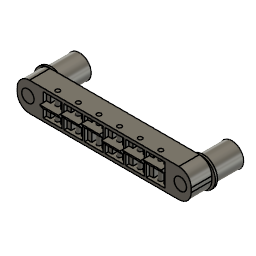
logo metal_ (Autodesk Fusion 360 archive; units mm, degrees)
design "Most Gotoh"
part number: 2026-09-04-10-43-11-082
Autodesk Fusion 360 part; units mm, degrees
note: some values were not read from the file. Chosen so that the rebuilt part matches the saved one: which bodies a step acts on; which face or edge a step refers to.
sketch "Szkic1" plane through (0, 0, 0) normal (0, 0, 1) x (1, 0, 0)
  line L0 (0, 0) -> (74, 0) construction
  circle A0 centre (0, 0) radius 3
  circle A1 centre (74, 0) radius 3
  line L1 (73.25, 7) -> (0.75, 7)
  line L2 (-5.25, 1) -> (-5.25, -1)
  line L3 (0.75, -7) -> (73.25, -7)
  line L4 (79.25, -1) -> (79.25, 1)
  line L5 (37, 5.5) -> (37, -5.5) construction
  line L6 (36.5, 5.5) -> (36.5, -5.5)
  line L7 (37.5, 5.5) -> (37.5, -5.5)
  line L8 (46.5, 5.5) -> (46.5, -5.5)
  line L9 (39.5, 5.5) -> (39.5, -5.5)
  line L10 (44.5, 5.5) -> (44.5, -5.5)
  line L11 (54.5, 5.5) -> (54.5, -5.5)
  line L12 (56.5, 5.5) -> (56.5, -5.5)
  line L13 (49.5, 5.5) -> (49.5, -5.5)
  line L14 (47.5, 5.5) -> (47.5, -5.5)
  line L15 (59.5, 5.5) -> (59.5, -5.5)
  line L16 (64.5, 5.5) -> (64.5, -5.5)
  line L17 (66.5, 5.5) -> (66.5, -5.5)
  line L18 (57.5, 5.5) -> (57.5, -5.5)
  line L19 (24.5, 5.5) -> (24.5, -5.5)
  line L20 (17.5, 5.5) -> (17.5, -5.5)
  line L21 (34.5, 5.5) -> (34.5, -5.5)
  line L22 (26.5, 5.5) -> (26.5, -5.5)
  line L23 (27.5, 5.5) -> (27.5, -5.5)
  line L24 (36.5, 5.5) -> (36.5, -5.5)
  line L25 (19.5, 5.5) -> (19.5, -5.5)
  line L26 (16.5, 5.5) -> (16.5, -5.5)
  line L27 (7.5, 5.5) -> (7.5, -5.5)
  line L28 (29.5, 5.5) -> (29.5, -5.5)
  line L29 (9.5, 5.5) -> (9.5, -5.5)
  line L30 (14.5, 5.5) -> (14.5, -5.5)
  arc A2 (79.25, 1) -> (73.25, 7) centre (73.25, 1) ccw
  arc A3 (73.25, -7) -> (79.25, -1) centre (73.25, -1) ccw
  arc A4 (-5.25, -1) -> (0.75, -7) centre (0.75, -1) ccw
  arc A5 (0.75, 7) -> (-5.25, 1) centre (0.75, 1) ccw
  line L31 (66.5, 5.5) -> (7.5, 5.5)
  line L32 (7.5, -5.5) -> (66.5, -5.5)
  point P0 (-5.25, 7)
  point P1 (-5.25, -7)
  point P2 (79.25, -7)
  point P3 (37, 0)
  dimension "d1" = 74
  dimension "d2" = 6
  dimension "d3" = 6
  dimension "d4" = 84.5
  dimension "d5" = 14
  dimension "d15" = -2
  dimension "d16" = 2
  dimension "d17" = -9
  dimension "d18" = -2
  dimension "d19" = 2
  dimension "d20" = -9
  dimension "d21" = -2
  dimension "d22" = 2
  dimension "d23" = 6
  dimension "d24" = 6
  constraint coincident L0.start A0.centre
  constraint horizontal L0
  constraint coincident L0.end A1.centre
  constraint perpendicular L1 L2
  constraint parallel L1 L3
  constraint parallel L2 L4
  constraint midpoint L0 P3
  constraint coincident L7.start L31
  constraint coincident L6.start L31
  constraint coincident L7.end L32
  constraint coincident L6.end L32
  constraint coincident L5.end L32
  constraint coincident L5.start L31
  constraint symmetric L5 L7.start L6.start
  constraint symmetric L5 L7.end L6.end
  constraint symmetric L5 L8.start L23.start
  constraint symmetric L5 L8.end L23.end
  constraint symmetric L5 L9.start L21.start
  constraint symmetric L5 L9.end L21.end
  constraint symmetric L5 L10.start L28.start
  constraint symmetric L5 L10.end L28.end
  constraint symmetric L5 L13.end L19.end
  constraint symmetric L5 L13.start L19.start
  constraint symmetric L5 L11.end L25.end
  constraint symmetric L5 L11.start L25.start
  constraint symmetric L5 L12.start L20.start
  constraint symmetric L5 L12.end L20.end
  constraint symmetric L5 L14.start L22.start
  constraint symmetric L5 L14.end L22.end
  constraint symmetric L5 L15.end L30.end
  constraint symmetric L5 L15.start L30.start
  constraint symmetric L5 L16.end L29.end
  constraint symmetric L5 L18.end L26.end
  constraint symmetric L5 L17.end L27.end
  constraint symmetric L5 L17.start L27.start
  constraint symmetric L5 L16.start L29.start
  constraint symmetric L5 L18.start L26.start
  constraint tangent L1 A2
  constraint tangent L4 A2
  constraint coincident P2 L4
  constraint coincident P2 L3
  constraint tangent L4 A3
  constraint tangent L3 A3
  constraint equal A2 A3
  constraint coincident P1 L3
  constraint coincident P1 L2
  constraint tangent L3 A4
  constraint tangent L2 A4
  constraint equal A2 A4
  constraint coincident P0 L1
  constraint coincident P0 L2
  constraint tangent L1 A5
  constraint tangent L2 A5
  measures "d1" distance of L0.start L0.end
  measures "d2" diameter of A0
  measures "d3" diameter of A1
  measures "d4" distance of P1 P2
  measures "d5" distance of P0 P1
  measures "d23" radius of A2
  measures "d24" radius of A5
extrude "Wyciągnięcie proste1" add sketch "Szkic1" against normal blind 10 contours L1 L2 L3 L4 A2 A3 A4 A5 | L6 L7 L24 L31 L32 | L6 L21 L24 L31 L32 | L7 L9 L31 L32 | L21 L28 L31 L32 | L9 L10 L31 L32 | L23 L28 L31 L32 | L8 L10 L31 L32 | L22 L23 L31 L32 | L8 L14 L31 L32 | L19 L22 L31 L32 | L13 L14 L31 L32 | L19 L25 L31 L32 | L11 L13 L31 L32 | L20 L25 L31 L32 | L11 L12 L31 L32 | L20 L26 L31 L32 | L12 L18 L31 L32 | L26 L30 L31 L32 | L15 L18 L31 L32 | L29 L30 L31 L32 | L15 L16 L31 L32 | L27 L29 L31 L32 | L16 L17 L31 L32 makes body 1
extrude "Wyciągnięcie proste2" cut sketch "Szkic1" against normal blind 8 contours L21 L28 L31 L32 | L9 L10 L31 L32 | L19 L25 L31 L32 | L11 L13 L31 L32 | L29 L30 L31 L32 | L15 L16 L31 L32 bodies 1
extrude "Wyciągnięcie proste3" cut sketch "Szkic1" against normal blind 1.5 contours L6 L21 L24 L31 L32 | L7 L9 L31 L32 | L23 L28 L31 L32 | L8 L10 L31 L32 | L19 L22 L31 L32 | L13 L14 L31 L32 | L20 L25 L31 L32 | L11 L12 L31 L32 | L26 L30 L31 L32 | L15 L18 L31 L32 | L27 L29 L31 L32 | L16 L17 L31 L32 bodies 1
sketch "Szkic2" plane through (0, -7, 0) normal (0, -1, 0) x (1, 0, 0)
  line L0 (73.25, 0) -> (0.75, 0)
  line L1 (0.75, 0) -> (0.75, -10)
  line L2 (0.75, -10) -> (73.25, -10)
  line L3 (73.25, -10) -> (73.25, 0)
  line L4 (37, 0) -> (37, -10)
  line L5 (27.5, 0) -> (36.5, 0)
  line L6 (36.5, 0) -> (36.5, -1.5)
  line L7 (36.5, -1.5) -> (34.5, -1.5)
  line L8 (34.5, -1.5) -> (34.5, -8)
  line L9 (34.5, -8) -> (29.5, -8)
  line L10 (29.5, -8) -> (29.5, -1.5)
  line L11 (29.5, -1.5) -> (27.5, -1.5)
  line L12 (27.5, -1.5) -> (27.5, 0)
  line L13 (17.5, 0) -> (26.5, 0)
  line L14 (26.5, 0) -> (26.5, -1.5)
  line L15 (26.5, -1.5) -> (24.5, -1.5)
  line L16 (24.5, -1.5) -> (24.5, -8)
  line L17 (24.5, -8) -> (19.5, -8)
  line L18 (19.5, -8) -> (19.5, -1.5)
  line L19 (19.5, -1.5) -> (17.5, -1.5)
  line L20 (17.5, -1.5) -> (17.5, 0)
  line L21 (7.5, 0) -> (16.5, 0)
  line L22 (16.5, 0) -> (16.5, -1.5)
  line L23 (16.5, -1.5) -> (14.5, -1.5)
  line L24 (14.5, -1.5) -> (14.5, -8)
  line L25 (14.5, -8) -> (9.5, -8)
  line L26 (9.5, -8) -> (9.5, -1.5)
  line L27 (9.5, -1.5) -> (7.5, -1.5)
  line L28 (7.5, -1.5) -> (7.5, 0)
  line L29 (37.5, 0) -> (46.5, 0)
  line L30 (46.5, 0) -> (46.5, -1.5)
  line L31 (46.5, -1.5) -> (44.5, -1.5)
  line L32 (44.5, -1.5) -> (44.5, -8)
  line L33 (44.5, -8) -> (39.5, -8)
  line L34 (39.5, -8) -> (39.5, -1.5)
  line L35 (39.5, -1.5) -> (37.5, -1.5)
  line L36 (37.5, -1.5) -> (37.5, 0)
  line L37 (47.5, 0) -> (56.5, 0)
  line L38 (56.5, 0) -> (56.5, -1.5)
  line L39 (56.5, -1.5) -> (54.5, -1.5)
  line L40 (54.5, -1.5) -> (54.5, -8)
  line L41 (54.5, -8) -> (49.5, -8)
  line L42 (49.5, -8) -> (49.5, -1.5)
  line L43 (49.5, -1.5) -> (47.5, -1.5)
  line L44 (47.5, -1.5) -> (47.5, 0)
  line L45 (57.5, 0) -> (66.5, 0)
  line L46 (66.5, 0) -> (66.5, -1.5)
  line L47 (66.5, -1.5) -> (64.5, -1.5)
  line L48 (64.5, -1.5) -> (64.5, -8)
  line L49 (64.5, -8) -> (59.5, -8)
  line L50 (59.5, -8) -> (59.5, -1.5)
  line L51 (59.5, -1.5) -> (57.5, -1.5)
  line L52 (57.5, -1.5) -> (57.5, 0)
  circle A0 centre (62, -2.5) radius 1
  circle A1 centre (52, -2.5) radius 1
  circle A2 centre (42, -2.5) radius 1
  circle A3 centre (32, -2.5) radius 1
  circle A4 centre (22, -2.5) radius 1
  circle A5 centre (12, -2.5) radius 1
  line L53 (96.0022, -7.6051) -> (91.0022, -7.6051)
  line L54 (91.0022, -7.6051) -> (91.0022, -1.3015)
  circle A6 centre (93.5022, -2.3015) radius 1
  line L55 (96.0022, -1.3015) -> (96.0022, -7.6051)
  line L56 (98.0022, -1.3015) -> (98.0022, 2.0377)
  line L57 (98.0022, 2.0377) -> (89.0022, 2.0377)
  line L58 (89.0022, 2.0377) -> (89.0022, -1.3015)
  line L59 (98.0022, -1.3015) -> (96.0022, -1.3015)
  line L60 (91.0022, -1.3015) -> (89.0022, -1.3015)
  circle A7 centre (12, -2.5) radius 1.5
  circle A8 centre (22, -2.5) radius 1.5
  circle A9 centre (32, -2.5) radius 1.5
  circle A10 centre (42, -2.5) radius 1.5
  circle A11 centre (52, -2.5) radius 1.5
  circle A12 centre (62, -2.5) radius 1.5
  dimension "d32" = 2
  dimension "d35" = -50
  dimension "d36" = 0
  dimension "d39" = 2
  dimension "d60" = 3
  dimension "d63" = 50
  dimension "d64" = 0
  constraint midpoint L0 L4.start
  constraint midpoint L2 L4.end
  constraint horizontal L57
  constraint perpendicular L56 L59
  constraint perpendicular L58 L60
  constraint concentric A5 A7
  measures "d32" diameter of A0
  measures "d39" diameter of A6
  measures "d60" diameter of A7
extrude "Wyciągnięcie proste4" cut sketch "Szkic2" against normal blind 20 contours A0 | A1 | A2 | A3 | A4 | A5 bodies 1
extrude "Wyciągnięcie proste5" add sketch "Szkic2" along normal blind 2 separate body contours L53 L54 L55 L56 L57 L58 L59 L60 makes body 2
sketch "Szkic3" plane through (98.0022, 0, 0) normal (1, 0, 0) x (0, 0, -1)
  line L0 (1.3015, -7) -> (-2.0377, -7)
  line L1 (-2.0377, -7) -> (-2.0377, -9)
  line L2 (-2.0377, -9) -> (1.3015, -9)
  line L3 (1.3015, -9) -> (1.3015, -7)
  line L4 (-2.0377, -7) -> (-0.7426, -9)
  constraint coincident L0.end L1.start
  constraint coincident L2 L4.end
extrude "Wyciągnięcie proste6" cut sketch "Szkic3" against normal blind 10 contours L1 L2 L4 bodies 2
extrude "Wyciągnięcie proste7" add sketch "Szkic2" against normal blind 14 separate body contours A0 | A1 | A2 | A3 | A4 | A5 makes body 3 at (32.6982, 2.3333, -1.7841) makes body 4 at (61.3018, 2.3333, -1.7841) makes body 5 at (22.995, 2.3333, -2.5996) makes body 6 at (41.3018, 2.3333, -1.7841) makes body 7 at (51.3018, 2.3333, -1.7841) makes body 8 at (12.995, 2.3333, -2.5996)
move_body "Przesuń1" bodies 2 to x (1, 0, 0) y (0, 1, 0) z (0, 0, 1) at (-31.5022, 2, -0.1985)
move_body "Przesuń2" bodies 2 to x (1, 0, 0) y (0, 1, 0) z (0, 0, 1) at (0, 8, 0)
pattern_linear "Szyk prostokątny1" count 6 spacing 10 along (-1, 0, 0) of bodies 2 makes body 9 at (51.9751, 3, 0.7252) makes body 10 at (41.9751, 3, 0.7252) makes body 11 at (31.9751, 3, 0.7252) makes body 12 at (21.9751, 3, 0.7252) makes body 13 at (11.9751, 3, 0.7252)
move_body "Przesuń3" bodies 9 to x (1, 0, 0) y (0, 1, 0) z (0, 0, 1) at (0, -1, 0)
move_body "Przesuń4" bodies 10 to x (1, 0, 0) y (0, 1, 0) z (0, 0, 1) at (0, -2, 0)
move_body "Przesuń5" bodies 12 to x (1, 0, 0) y (0, 1, 0) z (0, 0, 1) at (0, -1, 0)
move_body "Przesuń6" bodies 13 to x (1, 0, 0) y (0, 1, 0) z (0, 0, 1) at (0, -2, 0)
sketch "Szkic4" plane through (0, 0, -10) normal (0, 0, -1) x (-1, 0, 0)
  circle A0 centre (0, 0) radius 3
  circle A1 centre (-74, 0) radius 3
  line L0 (-0.75, 7) -> (-73.25, 7)
  line L1 (-79.25, 1) -> (-79.25, -1)
  line L2 (-73.25, -7) -> (-0.75, -7)
  line L3 (5.25, -1) -> (5.25, 1)
  circle A2 centre (0, 0) radius 3
  circle A3 centre (-74, 0) radius 3
  circle A4 centre (0, 0) radius 7
  circle A5 centre (-74, 0) radius 7
  circle A6 centre (0, 0) radius 5.75
  circle A7 centre (-74, 0) radius 5.75
  dimension "d50" = 14
  dimension "d51" = 14
  dimension "d52" = 11.5
  dimension "d53" = 11.5
  constraint concentric A2 A4
  constraint concentric A3 A5
  constraint concentric A4 A6
  constraint concentric A3 A7
  measures "d50" diameter of A4
  measures "d51" diameter of A5
  measures "d52" diameter of A6
  measures "d53" diameter of A7
extrude "Wyciągnięcie proste8" add sketch "Szkic4" against normal blind 10 separate body contours A0 A2 | A1 A3 makes body 14 at (-2.9963, -0.1495, -3.3333) makes body 15 at (75.3686, -2.6696, -6.6667)
extrude "Wyciągnięcie proste9" add sketch "Szkic4" along normal blind 1 separate body contours A4 | A5 | A6 | A7 makes body 16 at (-5.6294, -0.4968, -10) makes body 17 at (68.3594, -0.3478, -10)
extrude "Wyciągnięcie proste10" add sketch "Szkic4" along normal blind 15 contours A6 | A7 bodies 14 15 16 17
extrude "Wyciągnięcie proste11" add sketch "Szkic2" along normal blind 1.5 contours A0 | A1 | A2 | A3 | A4 | A5 | A7 | A8 | A9 | A10 | A11 | A12 bodies 3 4 5 6 7 8
fillet "Zaokrąglenie1" radius 0.5 6 edges at (30.6015, -8.5, -3.0424) (60.6015, -8.5, -3.0424) (20.6015, -8.5, -3.0424) (40.6015, -8.5, -3.0424) (50.6015, -8.5, -3.0424) (10.6015, -8.5, -3.0424) on bodies 3 4 5 6 7 8
named bodies: "Most", "Wozek", "Wozek (1)", "Wozek (2)", "Wozek (3)", "Wozek (4)", "Wozek (5)", "trzpien 1", "trzpien 2"

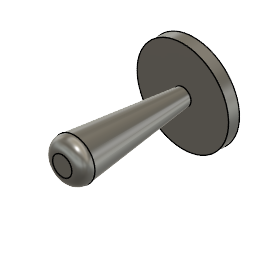
design "switch"
part number: 2026-09-05-00-23-10-023
Autodesk Fusion 360 part; units mm, degrees
sketch "Szkic1" plane through (0, 0, 0) normal (0, 0, 1) x (1, 0, 0)
  circle A0 centre (4170.9015, 1881.5344) radius 10
  line L0 (4170.898, 1886.1668) -> (4170.905, 1876.9019) construction
  arc A1 (4174.898, 1886.1698) -> (4171.0643, 1890.1634) centre (4170.898, 1886.1668) ccw construction
  line L1 (4166.8909, 1842.6943) -> (4166.8839, 1851.9378)
  arc A2 (4167.0998, 1876.917) -> (4171.3719, 1872.9292) centre (4171.0998, 1876.92) ccw construction
  circle A3 centre (4170.6925, 1847.3117) radius 6
  line L2 (4167.0998, 1876.917) -> (4167.0929, 1886.1605)
  arc A4 (4171.1629, 1838.7066) -> (4174.696, 1842.6823) centre (4170.696, 1842.6793) ccw
  line L3 (4174.689, 1851.9472) -> (4174.696, 1842.6823)
  line L4 (4170.689, 1851.9442) -> (4170.696, 1842.6793) construction
  circle A5 centre (4170.6925, 1847.3117) radius 10
  line L5 (4170.6925, 1850.8117) -> (4170.6925, 1843.8117) construction
  arc A6 (4170.8553, 1855.9407) -> (4166.8839, 1851.9378) centre (4170.8839, 1851.9408) ccw
  line L6 (4174.6925, 1850.8117) -> (4174.6925, 1843.8117)
  arc A7 (4174.689, 1851.9472) -> (4170.8553, 1855.9407) centre (4170.689, 1851.9442) ccw
  arc A8 (4166.8909, 1842.6943) -> (4171.1629, 1838.7066) centre (4170.8909, 1842.6973) ccw
  line L7 (4174.898, 1886.1698) -> (4174.905, 1876.9049)
  circle A9 centre (4170.9015, 1881.5344) radius 6
  arc A10 (4171.0643, 1890.1634) -> (4167.0929, 1886.1605) centre (4171.0929, 1886.1635) ccw construction
  arc A11 (4171.3719, 1872.9292) -> (4174.905, 1876.9049) centre (4170.905, 1876.9019) ccw construction
  circle A12 centre (4170.9015, 1881.5344) radius 8.3467
  circle A13 centre (4170.9015, 1881.5344) radius 1.5
  point P0 (4170.6925, 1847.3117)
  point P1 (4170.6925, 1847.3117)
  dimension "d2" = 4
  dimension "d3" = 20
  dimension "d4" = 12
  dimension "d5" = 20
  dimension "d6" = 12
  dimension "d36" = 4
  dimension "d44" = 3
  constraint parallel L2 L7
  constraint tangent L2 A10
  constraint tangent A1 L7
  constraint equal A1 A10
  constraint coincident A1.end A10.start
  constraint tangent L7 A11
  constraint equal A10 A11
  constraint tangent A2 L2
  constraint equal A2 A10
  constraint coincident L0.start A1.centre
  constraint coincident L0.end A11.centre
  constraint midpoint A0.centre L0
  constraint concentric A0 A9
  constraint midpoint P1 L5
  constraint concentric A3 A5
  constraint parallel L1 L3
  constraint tangent L1 A6
  constraint tangent L3 A7
  constraint equal A6 A7
  constraint coincident A6.start A7.end
  constraint tangent A4 L3
  constraint equal A4 A6
  constraint tangent L1 A8
  constraint equal A6 A8
  constraint coincident L4.start A7.centre
  constraint coincident A4.centre L4.end
  constraint midpoint P1 L4
  constraint concentric A9 A12
  constraint concentric A12 A13
  measures "d2" radius of A10
  measures "d3" diameter of A0
  measures "d4" diameter of A9
  measures "d5" diameter of A5
  measures "d6" diameter of A3
  measures "d36" radius of A6
  measures "d44" diameter of A13
extrude "Wyciągnięcie proste1" add sketch "Szkic1" against normal blind 2 contours A12
extrude "Wyciągnięcie proste2" add sketch "Szkic1" against normal blind 2 contours L7 A9 | L7 A9 | A13
ref_plane "Płaszczyzna konstrukcyjna1" through (4168.7371, 1881.5341, 22) normal (0, 0, 1) x (1, 0, 0)
sketch "Szkic2" plane through (0, 0, 22) normal (0, 0, 1) x (1, 0, 0)
  circle A0 centre (4170.9015, 1881.5344) radius 4
  point P0 (4170.9015, 1881.5344)
  dimension "d43" = 8
  constraint coincident P0 A0.centre
  measures "d43" diameter of A0
loft "Wyciągnięcie złożone1" add profiles "Szkic1", "Szkic2" section 1 contours A13 section 2
fillet "Zaokrąglenie1" radius 2 1 edges at (4167.1722, 1882.9808, 22)

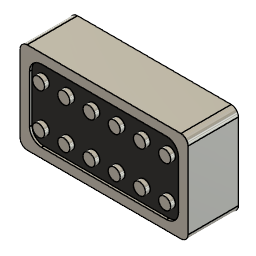
design "pickup"
part number: 2026-09-04-22-53-51-422
Autodesk Fusion 360 part; units mm, degrees
sketch "Szkic1" plane through (0, 0, 0) normal (0, 0, 1) x (1, 0, 0)
  line L0 (-22, 15) -> (42, 15)
  line L1 (45, 12) -> (45, -20)
  line L2 (42, -23) -> (-22, -23)
  line L3 (-25, -20) -> (-25, 12)
  arc A0 (-22, 15) -> (-25, 12) centre (-22, 12) ccw
  arc A1 (45, 12) -> (42, 15) centre (42, 12) ccw
  arc A2 (42, -23) -> (45, -20) centre (42, -20) ccw
  arc A3 (-25, -20) -> (-22, -23) centre (-22, -20) ccw
  arc A4 (44.5, 12) -> (42, 14.5) centre (42, 12) ccw
  line L4 (-22, 14.5) -> (42, 14.5)
  arc A5 (-22, 14.5) -> (-24.5, 12) centre (-22, 12) ccw
  line L5 (-24.5, -20) -> (-24.5, 12)
  arc A6 (-24.5, -20) -> (-22, -22.5) centre (-22, -20) ccw
  line L6 (42, -22.5) -> (-22, -22.5)
  arc A7 (42, -22.5) -> (44.5, -20) centre (42, -20) ccw
  line L7 (44.5, 12) -> (44.5, -20)
  line L8 (-16, 11) -> (36, 11)
  line L9 (-21, -14) -> (-21, 6)
  line L10 (36, -19) -> (-16, -19)
  line L11 (41, 6) -> (41, -14)
  arc A8 (41, 6) -> (36, 11) centre (36, 6) ccw
  arc A9 (36, -19) -> (41, -14) centre (36, -14) ccw
  arc A10 (-21, -14) -> (-16, -19) centre (-16, -14) ccw
  arc A11 (-16, 11) -> (-21, 6) centre (-16, 6) ccw
  line L12 (10, 15) -> (10, -23) construction
  line L13 (4.75, 15) -> (4.75, -23) construction
  line L14 (-21, 4.5) -> (42, 4.5) construction
  circle A12 centre (4.75, 4.5) radius 2.5
  line L15 (45, -4) -> (-24.5, -4) construction
  line L16 (34.5, -4) -> (-35, -4) construction
  circle A13 centre (-5.75, 4.5) radius 2.5
  line L17 (24, -4) -> (-45.5, -4) construction
  circle A14 centre (-16.25, 4.5) radius 2.5
  line L18 (45, -21) -> (-24.5, -21) construction
  circle A15 centre (4.75, -12.5) radius 2.5
  line L19 (34.5, -21) -> (-35, -21) construction
  circle A16 centre (-5.75, -12.5) radius 2.5
  line L20 (24, -21) -> (-45.5, -21) construction
  circle A17 centre (-16.25, -12.5) radius 2.5
  circle A18 centre (36.25, -12.5) radius 2.5
  circle A19 centre (36.25, 4.5) radius 2.5
  circle A20 centre (25.75, -12.5) radius 2.5
  circle A21 centre (25.75, 4.5) radius 2.5
  circle A22 centre (15.25, -12.5) radius 2.5
  circle A23 centre (15.25, 4.5) radius 2.5
  point P0 (-25, 15)
  point P1 (45, 15)
  point P2 (-25, -23)
  point P3 (20, 0)
  point P4 (36, 6)
  point P5 (36, -14)
  dimension "d1" = 70
  dimension "d2" = 38
  dimension "d3" = 3
  dimension "d4" = 0.5
  dimension "d6" = 5
  dimension "d11" = 5.25
  dimension "d13" = 5
  dimension "d16" = -21
  dimension "d17" = -17
  constraint horizontal L0
  constraint vertical L1
  constraint horizontal L2
  constraint vertical L3
  constraint coincident P0 L3
  constraint coincident P0 L0
  constraint tangent L3 A0
  constraint tangent L0 A0
  constraint coincident P1 L0
  constraint coincident P1 L1
  constraint tangent L0 A1
  constraint tangent L1 A1
  constraint equal A0 A1
  constraint tangent L2 A2
  constraint tangent L1 A2
  constraint equal A0 A2
  constraint coincident P2 L2
  constraint coincident P2 L3
  constraint tangent L2 A3
  constraint tangent L3 A3
  constraint equal A0 A3
  constraint tangent L8 A8
  constraint tangent L11 A8
  constraint tangent L11 A9
  constraint tangent L10 A9
  constraint equal A8 A9
  constraint tangent L10 A10
  constraint tangent L9 A10
  constraint equal A8 A10
  constraint tangent L9 A11
  constraint tangent L8 A11
  constraint equal A8 A11
  constraint midpoint L0 L12.start
  constraint midpoint L2 L12.end
  constraint coincident L9 L14.start
  constraint coincident L14 A12.centre
  constraint coincident L13 A12.centre
  constraint midpoint L1 L15.start
  constraint midpoint L5 L15.end
  constraint symmetric origin L12 P3
  constraint symmetric A10.centre L12 P5
  constraint symmetric A11.centre L12 P4
  constraint symmetric L12 A12 A23
  constraint symmetric L12 A13 A21
  constraint symmetric L12 A14 A19
  constraint symmetric L12 A15 A22
  constraint symmetric L12 A16 A20
  constraint symmetric L12 A17 A18
  measures "d1" distance of P0 P1
  measures "d2" distance of P0 P2
  measures "d3" radius of A0
  measures "d6" radius of A8
  measures "d13" diameter of A12
extrude "Wyciągnięcie proste1" add sketch "Szkic1" along normal blind 1 contours L0 L1 L2 L3 A0 A1 A2 A3 | A4 L4 A5 L5 A6 L6 A7 L7 makes body 1
extrude "Wyciągnięcie proste2" add sketch "Szkic1" against normal blind 20 contours L0 L1 L2 L3 A0 A1 A2 A3 bodies 1
extrude "Wyciągnięcie proste3" add sketch "Szkic1" against normal blind 1 separate body contours L8 L9 L10 L11 A8 A9 A10 A11 makes body 2
extrude "Wyciągnięcie proste4" add sketch "Szkic1" along normal blind 2 separate body contours A12 | A13 | A14 | A15 | A16 | A17 | A18 | A19 | A20 | A21 | A22 | A23 makes body 3 at (7.2469, -12.6246, 1.3333) makes body 4 at (38.7469, 4.3754, 1.3333) makes body 5 at (-3.2531, 4.3754, 1.3333) makes body 6 at (7.2469, 4.3754, 1.3333) makes body 7 at (38.7469, -12.6246, 1.3333) makes body 8 at (-3.2531, -12.6246, 1.3333) makes body 9 at (17.7469, -12.6246, 1.3333) makes body 10 at (28.2469, 4.3754, 1.3333) makes body 11 at (-13.7531, 4.3754, 1.3333) makes body 12 at (17.7469, 4.3754, 1.3333) makes body 13 at (28.2469, -12.6246, 1.3333) makes body 14 at (-13.7531, -12.6246, 1.3333)
equation "d11 = ( 10.5 / 2 ) * 1 mm"
named bodies: "ramka", "podstawa"
